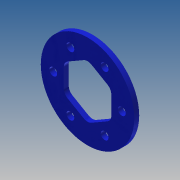
# Autodesk Inventor part: Wheel_external_hub_ring
Saved by Autodesk Inventor 2016 (Build 200138000, 138)
## iProperties
Created: 2014-05-28
Part Number: Wheel_external_hub_ring
Material: Aluminium 6061
Document SubType Name: Modeling
Designer: Yann
Density: 1 g/cm^3
Appearance: Bleu - Peinture murale - Brillant
d0: 60,000 mm
d4: 6,000 nd
d8: 3,175 mm
d9: 0,00 deg
d10: 22,000 mm
d11: 8,500 mm
d16: 3,500 mm
d21: 5,000 mm
d27: 1,000 mm
d28: 2,500 mm
d_profile_section: 40,000 mm
d_prfc_thickness: 3,000 mm
d_front_arm_od: 31,750 mm
d_front_arm_id: 29,261 mm
d_arm_length: 250,000 mm
d_suspension_height: 140,000 mm
d_aluminum_thickness: 3,175 mm
d_suspension_box_width: 40,000 mm
d_wheelbase: 1600,000 mm
a_tilt: 10,00 deg
d_rear_profile_width: 50,800 mm
d_rear_profile_height: 101,600 mm
d_central_profile_width: 50,800 mm
d_central_profile_height: 101,600 mm
d_handle_bar_od: 38,100 mm
d_handle_bar_id: 30,000 mm
a_direction_column: 35,00 deg
front_suspension_height: 140,930 mm
front_suspension_width: 150,000 mm
a_caster_angle: 25,00 deg
d_handlebar_arm_length: 80,000 mm
d_handlebar_pivot_offset: 65,000 mm
a_handlebar_angle: 60,00 deg
d_left_to_right_front_pivots: 28,000 mm
d_aluminum_bar_thickness: 12,700 mm
d_steering_arm_length: 70,000 mm
d_steering_height_from_hub_carrier_center: 18,000 mm
d6: 360,00 deg
Author: Yann
Autodesk Inventor part; units mm, degrees
ref_plane "YZ Plane" through (0, 0, 0) normal (1, 0, 0) x (0, 1, 0)
ref_plane "XZ Plane" through (0, 0, 0) normal (0, 1, 0) x (-1, 0, 0)
ref_plane "XY Plane" through (0, 0, 0) normal (0, 0, 1) x (1, 0, 0)
sketch "Esquisse1" plane through (0, 0, 0) normal (0, 1, 0) x (-1, 0, 0)
  line L0 (0, -42) -> (0, 42) construction
  circle A0 centre (0, 0) radius 30
  circle A1 centre (22, 0) radius 2.5
  circle A2 centre (11, 19.0526) radius 2.5
  circle A3 centre (-11, 19.0526) radius 2.5
  circle A4 centre (-22, 0) radius 2.5
  circle A5 centre (-11, -19.0526) radius 2.5
  circle A6 centre (11, -19.0526) radius 2.5
  line L1 (17.9263, -5.3263) -> (22, 0) construction
  line L2 (-2.5, -16.1785) -> (-12.761, -10.2543)
  line L3 (-15.261, -5.9242) -> (-15.261, 5.9242)
  line L4 (-12.761, 10.2543) -> (-2.5, 16.1785)
  line L5 (2.5, 16.1785) -> (12.761, 10.2543)
  line L6 (15.261, 5.9242) -> (15.261, -5.9242)
  line L7 (12.761, -10.2543) -> (2.5, -16.1785)
  arc A7 (2.5, 16.1785) -> (-2.5, 16.1785) centre (0, 11.8484) ccw
  arc A8 (15.261, 5.9242) -> (12.761, 10.2543) centre (10.261, 5.9242) ccw
  arc A9 (12.761, -10.2543) -> (15.261, -5.9242) centre (10.261, -5.9242) ccw
  arc A10 (-2.5, -16.1785) -> (2.5, -16.1785) centre (0, -11.8484) ccw
  arc A11 (-15.261, -5.9242) -> (-12.761, -10.2543) centre (-10.261, -5.9242) ccw
  arc A12 (-12.761, 10.2543) -> (-15.261, 5.9242) centre (-10.261, 5.9242) ccw
  line L8 (0, 0) -> (10.261, -5.9242) construction
  line L9 (22, 0) -> (0, 0) construction
  point P0 (0, -17.6219)
  point P1 (-15.261, -8.8109)
  point P2 (-15.261, 8.8109)
  point P3 (0, 17.6219)
  point P4 (15.261, 8.8109)
  point P5 (15.261, -8.8109)
  dimension "d0" = 60
  dimension "d6" = 360
  dimension "d10" = 22
  dimension "d21" = 5
  dimension "d30" = 5
  dimension "d31" = 30
  constraints: 18 end point, 13 centre point, 13 point on line, 12 point on circle, 12 tangent, 5 equal radius, 3 coincident, 1 parallel, 1 perpendicular, 26 other
  measures "d0" diameter of A0
  measures "d10" distance of point (0, 0) L1.end
  measures "d21" radius of A7
  measures "d30" diameter of A1
  measures "d31" angle of L9 L8
extrude "Extrusion1" add sketch "Esquisse1" against normal blind 3.175
equation "\"d8\" = d_aluminum_thickness"
equation "\"d_profile_section\" = 40"
equation "\"d_prfc_thickness\" = 3"
equation "\"d_front_arm_od\" = 31.75"
equation "\"d_front_arm_id\" = 29.2608"
equation "\"d_arm_length\" = 250"
equation "\"d_suspension_height\" = 140"
equation "\"d_aluminum_thickness\" = 3.175"
equation "\"d_suspension_box_width\" = 40"
equation "\"d_wheelbase\" = 1600"
equation "\"a_tilt\" = 10deg"
equation "\"d_rear_profile_width\" = 50.8"
equation "\"d_rear_profile_height\" = 101.6"
equation "\"d_central_profile_width\" = 50.8"
equation "\"d_central_profile_height\" = 101.6"
equation "\"d_handle_bar_od\" = 38.1"
equation "\"d_handle_bar_id\" = 30"
equation "\"a_direction_column\" = 35deg"
equation "\"front_suspension_height\" = 140.92977"
equation "\"front_suspension_width\" = 150"
equation "\"a_caster_angle\" = 25deg"
equation "\"d_handlebar_arm_length\" = 80"
equation "\"d_handlebar_pivot_offset\" = 65"
equation "\"a_handlebar_angle\" = 60deg"
equation "\"d_left_to_right_front_pivots\" = 28"
equation "\"d_aluminum_bar_thickness\" = 12.7"
equation "\"d_steering_arm_length\" = 70"
equation "\"d_steering_height_from_hub_carrier_center\" = 18"
equation "\"d_central_beam_inclination\" = 12"
equation "\"a_central_beam_inclination\" = 12deg"
equation "\"d_central_beam_screws_diameter\" = 8"
equation "\"d_rear_profile_wall_thickness\" = 4.7625"
equation "\"d_rear_profile_wall_thickness_1\" = 4.7625"
equation "\"d_central_pivot_screw_diameter\" = 15.875"
